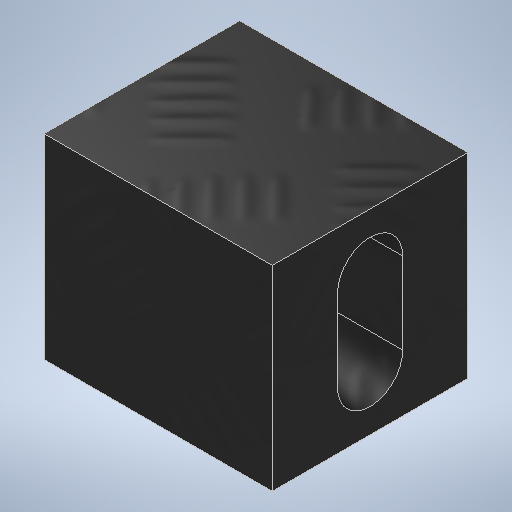
# Autodesk Inventor part: multiblock_12x12x14
Saved by Autodesk Inventor 2025.4 (Build 294407000, 407)
## iProperties
Created: 2026-06-08
Part Number: multiblock_12x12x14
Material: 폴리스티렌
Document SubType Name: Modeling
Designer: dalbi
Density: 1.021 g/cm^3
Appearance: 다이아몬드 플레이트 - 진회색
Mass: 1.59283 g
Surface Area: 12.108 cm^2
Volume: 1.56007 cm^3
Author: dalbi
Autodesk Inventor part; units mm, degrees
ref_plane "YZ Plane" through (0, 0, 0) normal (1, 0, 0) x (0, 1, 0)
ref_plane "XZ Plane" through (0, 0, 0) normal (0, 1, 0) x (-1, 0, 0)
ref_plane "XY Plane" through (0, 0, 0) normal (0, 0, 1) x (1, 0, 0)
sketch "스케치1" plane through (0, 0, 0) normal (0, 1, 0) x (-1, 0, 0)
  line L0 (7, 6) -> (-7, 6)
  line L1 (-7, 6) -> (-7, -6)
  line L2 (-7, -6) -> (7, -6)
  line L3 (7, -6) -> (7, 6)
  line L4 (7, 6) -> (-7, -6) construction
  line L5 (-7, 6) -> (7, -6) construction
  point P0 (0, 0)
  dimension "d0" = 14
  dimension "d1" = 12
  constraints: 12 end point, 2 midpoint, 2 parallel, 1 horizontal, 1 perpendicular
  measures "d0" distance of L0.start L0.end
  measures "d1" distance of L2.end L0.start
extrude "돌출1" add sketch "스케치1" along normal mid plane 12
sketch "스케치3" plane through (7, -6, -6) normal (1, 0, 0) x (0, 0, -1)
  line L0 (-14.9639, 6) -> (4.1102, 6) construction
  line L1 (-6, -0.8058) -> (-6, 13.755)
  line L2 (-12, 12) -> (0, 12) projected
  line L3 (-14.4911, 8.5) -> (7.0888, 8.5)
  arc A0 (-4, 8.5) -> (-8, 8.5) centre (-6, 8.5) ccw
  arc A1 (-8, 3.5) -> (-4, 3.5) centre (-6, 3.5) ccw
  line L4 (-8, 3.5) -> (-8, 8.5)
  line L5 (-4, 3.5) -> (-4, 8.5)
  point P0 (-6, 6)
  dimension "d8" = 6
  dimension "d9" = 5
  dimension "d10" = 4
  constraints: 10 end point, 4 point on circle, 4 point on line, 2 centre point, 2 horizontal, 1 symmetric about line, 1 vertical, 1 other
  measures "d8" distance between parallel lines of L2 L0
  measures "d9" diameter of L3 L0
  measures "d10" diameter of A0
extrude "돌출2" cut sketch "스케치3" against normal up to surface (14 mm away)
